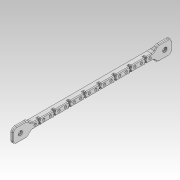
# Autodesk Inventor part: DoubleSolenoidBracket
Saved by Autodesk Inventor 2020 (Build 240168000, 168)
## iProperties
Created: 2021-09-21
Part Number: DoubleSolenoidBracket
Material: Generic
Document SubType Name: Modeling
Designer: DDeGo
Density: 1 g/cm^3
Appearance: Default
Author: DDeGo
Autodesk Inventor part; units mm, degrees
ref_plane "YZ Plane" through (0, 0, 0) normal (1, 0, 0) x (0, 1, 0)
ref_plane "XZ Plane" through (0, 0, 0) normal (0, 1, 0) x (-1, 0, 0)
ref_plane "XY Plane" through (0, 0, 0) normal (0, 0, 1) x (1, 0, 0)
sketch "Sketch1" plane through (0, 0, 0) normal (1, 0, 0) x (0, 1, 0)
  line L0 (0, 0) -> (8, 0)
  line L1 (8, 0) -> (8, -169)
  line L2 (8, -169) -> (0, -169)
  line L3 (0, -169) -> (0, 0)
  line L4 (4, 0) -> (4, -5) construction
  line L5 (4, -5) -> (4, -17) construction
  circle A0 centre (4, -5) radius 1.75
  circle A1 centre (4, -17) radius 1.75
  line L6 (2.75, -12) -> (2.75, -10) construction
  line L7 (5.25, -10) -> (5.25, -12) construction
  line L8 (8, -12) -> (5.25, -12) construction
  line L9 (2.75, -12) -> (0, -12) construction
  line L10 (0, -10) -> (2.75, -10) construction
  line L11 (5.25, -10) -> (8, -10) construction
  line L12 (5.25, -11) -> (2.75, -11) construction
  circle A2 centre (4, -38) radius 1.75
  line L13 (2.75, -33) -> (2.75, -31) construction
  line L14 (5.25, -31) -> (5.25, -33) construction
  circle A3 centre (4, -26) radius 1.75
  line L15 (4, -26) -> (4, -38) construction
  circle A4 centre (4, -59) radius 1.75
  line L16 (2.75, -54) -> (2.75, -52) construction
  line L17 (5.25, -52) -> (5.25, -54) construction
  circle A5 centre (4, -47) radius 1.75
  line L18 (4, -47) -> (4, -59) construction
  circle A6 centre (4, -80) radius 1.75
  line L19 (2.75, -75) -> (2.75, -73) construction
  line L20 (5.25, -73) -> (5.25, -75) construction
  circle A7 centre (4, -68) radius 1.75
  line L21 (4, -68) -> (4, -80) construction
  circle A8 centre (4, -101) radius 1.75
  line L22 (2.75, -96) -> (2.75, -94) construction
  line L23 (5.25, -94) -> (5.25, -96) construction
  circle A9 centre (4, -89) radius 1.75
  line L24 (4, -89) -> (4, -101) construction
  circle A10 centre (4, -122) radius 1.75
  line L25 (2.75, -117) -> (2.75, -115) construction
  line L26 (5.25, -115) -> (5.25, -117) construction
  circle A11 centre (4, -110) radius 1.75
  line L27 (4, -110) -> (4, -122) construction
  circle A12 centre (4, -143) radius 1.75
  line L28 (2.75, -138) -> (2.75, -136) construction
  line L29 (5.25, -136) -> (5.25, -138) construction
  circle A13 centre (4, -131) radius 1.75
  line L30 (4, -131) -> (4, -143) construction
  circle A14 centre (4, -164) radius 1.75
  line L31 (2.75, -159) -> (2.75, -157) construction
  line L32 (5.25, -157) -> (5.25, -159) construction
  circle A15 centre (4, -152) radius 1.75
  line L33 (4, -152) -> (4, -164) construction
  point P0 (4, -11)
  point P1 (5.25, -32)
  point P2 (2.75, -32)
  point P3 (4, -32)
  point P4 (5.25, -53)
  point P5 (2.75, -53)
  point P6 (4, -53)
  point P7 (5.25, -74)
  point P8 (2.75, -74)
  point P9 (4, -74)
  point P10 (5.25, -95)
  point P11 (2.75, -95)
  point P12 (4, -95)
  point P13 (5.25, -116)
  point P14 (2.75, -116)
  point P15 (4, -116)
  point P16 (5.25, -137)
  point P17 (2.75, -137)
  point P18 (4, -137)
  point P19 (5.25, -158)
  point P20 (2.75, -158)
  point P21 (4, -158)
  dimension "d0" = 12
  dimension "d1" = 3.5
  dimension "d2" = 5
  dimension "d3" = 2.5
  dimension "d4" = 2
  dimension "d5" = 8
  dimension "d8" = 21
  dimension "d13" = 5
  constraints: 68 end point, 16 centre point, 16 coincident, 10 perpendicular, 5 midpoint, 5 point on line, 3 parallel, 2 collinear, 1 equal radius, 1 horizontal, 1 vertical, 111 other
  measures "d0" distance of L4.end L5.end
  measures "d1" diameter of A0
  measures "d2" distance of L4.start L4.end
  measures "d3" distance between parallel lines of L6 L7
  measures "d4" distance of L7.start L7.end
  measures "d5" distance between parallel lines of L3 L1
  measures "d8" distance of A1.centre A2.centre
  measures "d13" distance from line of A14.centre L2
extrude "Extrusion1" add sketch "Sketch1" along normal blind 7
sketch "Sketch2" plane through (7, 0, 0) normal (1, 0, 0) x (0, 0, -1)
  circle A0 centre (5, 4) radius 1.75 construction
  circle A1 centre (17, 4) radius 1.75 construction
  line L0 (5, 4) -> (17, 4) construction
  line L1 (10.25, 2.75) -> (11.75, 2.75)
  line L2 (11.75, 2.75) -> (11.75, 5.25) construction
  line L3 (11.75, 5.25) -> (10.25, 5.25)
  line L4 (10.25, 5.25) -> (10.25, 2.75) construction
  line L5 (10.25, 2.75) -> (11.75, 5.25) construction
  line L6 (11.75, 2.75) -> (10.25, 5.25) construction
  line L7 (10.25, 5.25) -> (10.25, 8)
  line L8 (169, 8) -> (0, 8) construction
  line L9 (11.75, 5.25) -> (11.75, 8)
  line L10 (10.25, 8) -> (11.75, 8)
  line L11 (11.75, 2.75) -> (11.75, 0)
  line L12 (0, 0) -> (169, 0) construction
  line L13 (10.25, 2.75) -> (10.25, 0)
  line L14 (11.75, 0) -> (10.25, 0)
  point P0 (11, 4)
  dimension "d16" = 2.5
  dimension "d17" = 1.5
  constraints: 26 end point, 6 point on line, 3 midpoint, 3 parallel, 3 perpendicular, 2 horizontal, 1 vertical
  measures "d16" distance between parallel lines of L1 L3
  measures "d17" distance between parallel lines of L4 L2
extrude "Extrusion2" cut sketch "Sketch2" against normal blind 3.5
fillet "Fillet1" radius 1 4 edges at (5.25, 8, -10.25) (5.25, 8, -11.75) (5.25, 0, -10.25) (5.25, 0, -11.75)
fillet "Fillet1" radius 0.5 4 edges at (5.25, 2.75, -10.25) (5.25, 2.75, -11.75) (5.25, 5.25, -10.25) (5.25, 5.25, -11.75)
sketch "Sketch4" plane through (0, 0, 0) normal (-1, 0, 0) x (0, 0, 1)
  circle A0 centre (-5, 4) radius 1.75 projected
  circle A1 centre (-5, 4) radius 3
  circle A2 centre (-17, 4) radius 1.75 projected
  circle A3 centre (-17, 4) radius 3
  point P0 (0, 0)
  dimension "d25" = 6
  constraints: 2 centre point, 2 coincident, 1 equal radius
  measures "d25" diameter of A1
extrude "Extrusion4" cut sketch "Sketch4" against normal blind 3 contours A0 | A1 | A2 | A3
pattern_linear "Rectangular Pattern1" count 8 spacing 21 along (0, 0, -1) of "Extrusion4", "Extrusion2", "Fillet1"
ref_plane "Work Plane1" through (0, 0, -84.5) normal (0, 0, 1) x (1, 0, 0)
sketch "Sketch5" plane through (7, 0, 0) normal (1, 0, 0) x (0, 0, -1)
  line L0 (0, 0) -> (169, 0) construction
  line L1 (169, 8) -> (0, 8) construction
  line L2 (0, 0) -> (0, 8)
  line L3 (0, 8) -> (-5.5, 14)
  line L4 (-5.5, 14) -> (-25.5, 14)
  line L5 (-25.5, 14) -> (-25.5, -6)
  line L6 (-25.5, -6) -> (-5.5, -6)
  line L7 (-5.5, -6) -> (-5.5, 14) construction
  line L8 (0, 8) -> (0, 0) projected
  line L9 (-5.5, -6) -> (0, 0)
  line L10 (-5.5, 4) -> (-25.5, 4) construction
  circle A0 centre (-15.5, 4) radius 3
  line L11 (84.5, -10) -> (84.5, 18) projected
  dimension "d31" = 6
  dimension "d32" = 20
  dimension "d33" = 100
  dimension "d34" = 20
  constraints: 16 end point, 5 perpendicular, 3 midpoint, 1 centre point, 1 equal length
  measures "d31" diameter of A0
  measures "d32" distance of L4.end L5.end
  measures "d33" distance from line of L11 A0.centre
  measures "d34" distance of L3.end L4.end
extrude "Extrusion5" add sketch "Sketch5" against normal blind 3
mirror "Mirror1" about plane through (0, 0, -84.5) normal (0, 0, 1) of "Extrusion5"
fillet "Fillet2" radius 5 4 edges at (5.5, 14, 25.5) (5.5, -6, 25.5) (5.5, 14, -194.5) (5.5, -6, -194.5)
fillet "Fillet2" radius 5 8 edges at (5.5, 14, 5.5) (5.5, 0, 0) (5.5, 8, 0) (5.5, -6, 5.5) (5.5, 14, -174.5) (5.5, 8, -169) (5.5, 0, -169) (5.5, -6, -174.5)
chamfer "Chamfer1" distance 4 angle 45 2 edges at (4, 4, 0) (4, 4, -169)
fillet "Fillet3" radius 5 2 edges at (4, 4, 3.9999) (4, 4, -172.9999)
fillet "Fillet4" radius 1 152 edges at (7, 0.2929, -12.0429) (7, 0, -21.5) (7, 0.2929, -30.9571) (7, 1.625, -31.25) (7, 2.6036, -31.3964) (7, 2.75, -32) (7, 2.6036, -32.6036) (7, 1.625, -32.75) (7, 0.2929, -33.0429) (7, 0, -42.5) (7, 0.2929, -51.9571) (7, 1.625, -52.25) (7, 2.6036, -52.3964) (7, 2.75, -53) (7, 2.6036, -53.6036) (7, 1.625, -53.75) (7, 0.2929, -54.0429) (7, 0, -63.5) (7, 0.2929, -72.9571) (7, 1.625, -73.25) (7, 2.6036, -73.3964) (7, 2.75, -74) (7, 2.6036, -74.6036) (7, 1.625, -74.75) (7, 0.2929, -75.0429) (7, 0, -84.5) (7, 0.2929, -93.9571) (7, 1.625, -94.25) (7, 2.6036, -94.3964) (7, 2.75, -95) (7, 2.6036, -95.6036) (7, 1.625, -95.75) (7, 0.2929, -96.0429) (7, 0, -105.5) (7, 0.2929, -114.9571) (7, 1.625, -115.25) (7, 2.6036, -115.3964) (7, 2.75, -116) (7, 2.6036, -116.6036) (7, 1.625, -116.75) (7, 0.2929, -117.0429) (7, 0, -126.5) (7, 0.2929, -135.9571) (7, 1.625, -136.25) (7, 2.6036, -136.3964) (7, 2.75, -137) (7, 2.6036, -137.6036) (7, 1.625, -137.75) (7, 0.2929, -138.0429) (7, 0, -147.5) (7, 0.2929, -156.9571) (7, 1.625, -157.25) (7, 2.6036, -157.3964) (7, 2.75, -158) (7, 2.6036, -158.6036) (7, 1.625, -158.75) (7, 0.2929, -159.0429) (7, 0, -163.2752) (7, -0.4233, -168.8138) (7, -3, -171.75) (7, -5.5767, -174.6862) (7, -6, -183.0998) (7, -4.5355, -193.0355) (7, 4, -194.5) (7, 12.5355, -193.0355) (7, 14, -183.0998) (7, 13.5767, -174.6862) (7, 11, -171.75) (7, 8.4233, -168.8138) (7, 8, -163.2752) (7, 7.7071, -159.0429) (7, 6.375, -158.75) (7, 5.3964, -158.6036) (7, 5.25, -158) (7, 5.3964, -157.3964) (7, 6.375, -157.25) (7, 7.7071, -156.9571) (7, 8, -147.5) (7, 7.7071, -138.0429) (7, 6.375, -137.75) (7, 5.3964, -137.6036) (7, 5.25, -137) (7, 5.3964, -136.3964) (7, 6.375, -136.25) (7, 7.7071, -135.9571) (7, 8, -126.5) (7, 7.7071, -117.0429) (7, 6.375, -116.75) (7, 5.3964, -116.6036) (7, 5.25, -116) (7, 5.3964, -115.3964) (7, 6.375, -115.25) (7, 7.7071, -114.9571) (7, 8, -105.5) (7, 7.7071, -96.0429) (7, 6.375, -95.75) (7, 5.3964, -95.6036) (7, 5.25, -95) (7, 5.3964, -94.3964) (7, 6.375, -94.25) (7, 7.7071, -93.9571) (7, 8, -84.5) (7, 7.7071, -75.0429) (7, 6.375, -74.75) (7, 5.3964, -74.6036) (7, 5.25, -74) (7, 5.3964, -73.3964) (7, 6.375, -73.25) (7, 7.7071, -72.9571) (7, 8, -63.5) (7, 7.7071, -54.0429) (7, 6.375, -53.75) (7, 5.3964, -53.6036) (7, 5.25, -53) (7, 5.3964, -52.3964) (7, 6.375, -52.25) (7, 7.7071, -51.9571) (7, 8, -42.5) (7, 7.7071, -33.0429) (7, 6.375, -32.75) (7, 5.3964, -32.6036) (7, 5.25, -32) (7, 5.3964, -31.3964) (7, 6.375, -31.25) (7, 7.7071, -30.9571) (7, 8, -21.5) (7, 7.7071, -12.0429) (7, 6.375, -11.75) (7, 5.3964, -11.6036) (7, 5.25, -11) (7, 5.3964, -10.3964) (7, 6.375, -10.25) (7, 7.7071, -9.9571) (7, 8, -5.7248) (7, 8.4233, -0.1862) (7, 11, 2.75) (7, 13.5767, 5.6862) (7, 14, 14.0998) (7, 12.5355, 24.0355) (7, 4, 25.5) (7, -4.5355, 24.0355) (7, -6, 14.0998) (7, -5.5767, 5.6862) (7, -3, 2.75) (7, -0.4233, -0.1862) (7, 0, -5.7248) (7, 0.2929, -9.9571) (7, 1.625, -10.25) (7, 2.6036, -10.3964) (7, 2.75, -11) (7, 2.6036, -11.6036) (7, 1.625, -11.75)
equation "\"d13\" = d2"
equation "\"d30\" = d8"
body "Solid1"
